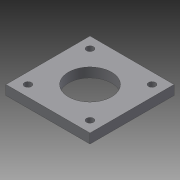
# Autodesk Inventor part: Vertical_Lead_Screw_Shaft_Mount_Plate_End
Saved by Autodesk Inventor 2015 (Build 190159000, 159)
## iProperties
Created: 2014-12-22
Part Number: Vertical_Lead_Screw_Shaft_Mount_Plate_End
Material: Generic
Document SubType Name: Modeling
Designer: Drew
Density: 1 g/cm^3
Appearance: Default
Author: Drew
Autodesk Inventor part; units mm, degrees
ref_plane "YZ Plane" through (0, 0, 0) normal (1, 0, 0) x (0, 1, 0)
ref_plane "XZ Plane" through (0, 0, 0) normal (0, 1, 0) x (-1, 0, 0)
ref_plane "XY Plane" through (0, 0, 0) normal (0, 0, 1) x (1, 0, 0)
sketch "Sketch1" plane through (0, 0, 0) normal (0, 1, 0) x (-1, 0, 0)
  line L0 (-21, -21) -> (21, -21)
  line L1 (21, -21) -> (21, 21)
  line L2 (21, 21) -> (-21, 21)
  line L3 (-21, 21) -> (-21, -21)
  line L4 (-21, -21) -> (21, 21) construction
  line L5 (21, -21) -> (-21, 21) construction
  circle A0 centre (15.5, 15.5) radius 1.75
  circle A1 centre (0, 0) radius 10.75
  line L6 (34.796, 0) -> (-29.6686, 0)
  line L7 (0, -38.1967) -> (0, 38.2612)
  circle A2 centre (15.5, -15.5) radius 1.75
  circle A3 centre (-15.5, 15.5) radius 1.75
  circle A4 centre (-15.5, -15.5) radius 1.75
  dimension "d0" = 42
  dimension "d1" = 42
  dimension "d4" = 3.5
  dimension "d8" = 21.5
  dimension "d13" = 31
  constraints: 16 end point, 5 centre point, 3 symmetric about line, 2 horizontal, 2 midpoint, 2 parallel, 1 coincident, 1 perpendicular, 1 point on line, 1 vertical, 3 other
  measures "d0" distance of L0.end L1.end
  measures "d1" distance of L1.end L2.end
  measures "d4" diameter of A0
  measures "d8" diameter of A1
  measures "d13" distance of A2.centre A0.centre
extrude "Extrusion4" add sketch "Sketch1" along normal blind 4.7625 contours L3 L6 A1 L7 L0 | L7 A1 L6 L1 L0 | L3 L2 L7 A1 L6 | L6 A1 L7 L2 L1
equation "\"d0\" = d1"
body "Solid4"
